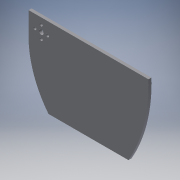
# Autodesk Inventor part: Bucket - door
Saved by Autodesk Inventor 2016 (Build 200138000, 138)
## iProperties
Created: 2015-12-17
Part Number: Bucket - door
Material: PET Plastic
Document SubType Name: Modeling
Designer: TimB
Density: 1.541 g/cm^3
Appearance: Polycarbonate - Clear
Author: TimB
Autodesk Inventor part; units mm, degrees
ref_plane "YZ Plane" through (0, 0, 0) normal (1, 0, 0) x (0, 1, 0)
ref_plane "XZ Plane" through (0, 0, 0) normal (0, 1, 0) x (-1, 0, 0)
ref_plane "XY Plane" through (0, 0, 0) normal (0, 0, 1) x (1, 0, 0)
sketch "Sketch1" plane through (0, 0, 0) normal (0, 0, 1) x (1, 0, 0)
  line L0 (-76.2, 50.8) -> (76.2, 50.8)
  line L1 (76.2, -50.8) -> (-76.2, 50.8) construction
  line L2 (-76.2, -50.8) -> (76.2, 50.8) construction
  line L3 (-76.2, 50.8) -> (-76.2, 25.4)
  arc A0 (-76.2, 25.4) -> (-50.8, -50.8) centre (42.7352, 22.7117) ccw
  arc A1 (50.8, -50.8) -> (76.2, 50.8) centre (-114.5506, 44.5126) ccw
  line L4 (-50.8, -50.8) -> (50.8, -50.8)
  point P0 (0, 0)
  dimension "d0" = 152.4
  dimension "d1" = 101.6
  dimension "d2" = 25.4
  dimension "d3" = 25.4
  dimension "d4" = 25.4
  constraints: 10 end point, 4 point on circle, 2 centre point, 2 midpoint, 1 horizontal
  measures "d0" distance of L0.start L0.end
  measures "d1" distance of L2.start L0.start
  measures "d2" distance of L0.start L3.end
  measures "d3" distance of L2.start L4.start
  measures "d4" distance of L1.start L4.end
extrude "Extrusion1" add sketch "Sketch1" along normal blind 3.81
sketch "Sketch2" plane through (0, 0, 3.81) normal (0, 0, 1) x (1, 0, 0)
  circle A0 centre (-60.12, 42.72) radius 1.75 projected
  circle A1 centre (-52.12, 34.72) radius 1.75 projected
  circle A2 centre (-68.12, 34.72) radius 1.75 projected
  circle A3 centre (-60.12, 26.72) radius 1.75 projected
  circle A4 centre (-60.12, 34.72) radius 2.85 projected
  point P0 (0, 0)
hole "Hole1" at (-60.12, 42.72, 3.81) at (-68.12, 34.72, 3.81) at (-60.12, 26.72, 3.81) at (-52.12, 34.72, 3.81) direction (0, 0, -1) diameter 3.7 end through all
sketch "Sketch3" plane through (0, 0, 3.81) normal (0, 0, 1) x (1, 0, 0)
  circle A0 centre (-60.12, 34.72) radius 2.85 projected
  point P0 (0, 0)
hole "Hole2" at (-60.12, 34.72, 3.81) direction (0, 0, -1) diameter 6 end through all
body "Solid1"
